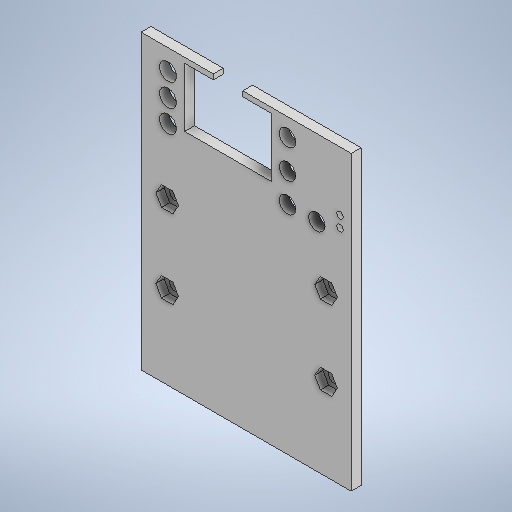
# Autodesk Inventor part: TES_Controller_V1_Case_Top
Saved by Autodesk Inventor 2025 (Build 290162000, 162)
## iProperties
Created: 2025-08-31
Part Number: TES_Controller_V1_Case_Top
Material: 常规
Document SubType Name: Modeling
Designer: 95052
Density: 1 g/cm^3
Appearance: 默认
Author: 95052
Autodesk Inventor part; units mm, degrees
ref_plane "YZ Plane" through (0, 0, 0) normal (1, 0, 0) x (0, 1, 0)
ref_plane "XZ Plane" through (0, 0, 0) normal (0, 1, 0) x (-1, 0, 0)
ref_plane "XY Plane" through (0, 0, 0) normal (0, 0, 1) x (1, 0, 0)
sketch "草图22" plane through (0, 0, 0) normal (0, 0, 1) x (1, 0, 0)
  line L0 (32.055, -44.6465) -> (-32.055, -44.6465)
  line L1 (-32.055, -44.6465) -> (-32.055, 44.6465)
  line L2 (-32.055, 44.6465) -> (32.055, 44.6465)
  line L3 (32.055, 44.6465) -> (32.055, -44.6465)
  line L4 (32.055, -44.6465) -> (-32.055, 44.6465) construction
  line L5 (-32.055, -44.6465) -> (32.055, 44.6465) construction
  line L6 (24.394, -19.5595) -> (-24.107, -19.5595) construction
  line L7 (-24.107, -19.5595) -> (-24.107, 4.4405) construction
  line L8 (-24.107, 4.4405) -> (24.394, 4.4405) construction
  line L9 (24.394, 4.4405) -> (24.394, -19.5595) construction
  line L10 (24.394, -19.5595) -> (-24.107, 4.4405) construction
  line L11 (-24.107, -19.5595) -> (24.394, 4.4405) construction
  circle A0 centre (-24.107, 4.4405) radius 1.7
  circle A1 centre (-24.107, -19.5595) radius 1.7
  circle A2 centre (24.394, -19.5595) radius 1.7
  circle A3 centre (24.394, 4.4405) radius 1.7
  point P0 (0, 0)
  point P1 (-14.525, 44.6465)
  point P2 (3.476, 44.6465)
  point P3 (0.1435, -7.5595)
  dimension "d101" = 89.293
  dimension "d102" = 64.11
  dimension "d103" = 7.661
  dimension "d104" = 7.948
  dimension "d105" = 25.087
  dimension "d106" = 40.206
  dimension "d107" = 17.53
  dimension "d108" = 28.579
  dimension "d109" = 3.4
  dimension "d110" = 3.4
  dimension "d111" = 3.4
  dimension "d112" = 3.4
  constraints: 24 end point, 4 centre point, 4 coincident, 4 midpoint, 4 parallel, 2 horizontal, 2 perpendicular, 2 point on line
  measures "d101" distance of L2.end L0.start
  measures "d102" distance of L0.start L0.end
  measures "d103" distance between parallel lines of L3 L9
  measures "d104" distance between parallel lines of L1 L7
  measures "d105" distance between parallel lines of L0 L6
  measures "d106" distance between parallel lines of L2 L8
  measures "d107" distance from line of L1 point (-14.525, 44.646)
  measures "d108" distance from line of L3 point (3.476, 44.646)
  measures "d109" diameter of A0
  measures "d110" diameter of A1
  measures "d111" diameter of A2
  measures "d112" diameter of A3
extrude "拉伸18" add sketch "草图22" along normal blind 0.5
sketch "草图23" plane through (0, 0, 0.5) normal (0, 0, 1) x (1, 0, 0)
  circle A0 centre (-24.107, 4.4405) radius 1.7 projected
  circle A1 centre (24.394, 4.4405) radius 1.7 projected
  circle A2 centre (24.394, -19.5595) radius 1.7 projected
  circle A3 centre (-24.107, -19.5595) radius 1.7 projected
  line L0 (-22.3749, -16.5595) -> (-20.6429, -19.5595)
  line L1 (-20.6429, -19.5595) -> (-22.3749, -22.5595)
  line L2 (-22.3749, -22.5595) -> (-25.8391, -22.5595)
  line L3 (-25.8391, -22.5595) -> (-27.5711, -19.5595)
  line L4 (-27.5711, -19.5595) -> (-25.8391, -16.5595)
  line L5 (-25.8391, -16.5595) -> (-22.3749, -16.5595)
  line L6 (-25.8391, 1.4405) -> (-27.5711, 4.4405)
  line L7 (-27.5711, 4.4405) -> (-25.8391, 7.4405)
  line L8 (-25.8391, 7.4405) -> (-22.3749, 7.4405)
  line L9 (-22.3749, 7.4405) -> (-20.6429, 4.4405)
  line L10 (-20.6429, 4.4405) -> (-22.3749, 1.4405)
  line L11 (-22.3749, 1.4405) -> (-25.8391, 1.4405)
  line L12 (22.6619, 1.4405) -> (20.9299, 4.4405)
  line L13 (20.9299, 4.4405) -> (22.6619, 7.4405)
  line L14 (22.6619, 7.4405) -> (26.1261, 7.4405)
  line L15 (26.1261, 7.4405) -> (27.8581, 4.4405)
  line L16 (27.8581, 4.4405) -> (26.1261, 1.4405)
  line L17 (26.1261, 1.4405) -> (22.6619, 1.4405)
  line L18 (22.6619, -22.5595) -> (20.9299, -19.5595)
  line L19 (20.9299, -19.5595) -> (22.6619, -16.5595)
  line L20 (22.6619, -16.5595) -> (26.1261, -16.5595)
  line L21 (26.1261, -16.5595) -> (27.8581, -19.5595)
  line L22 (27.8581, -19.5595) -> (26.1261, -22.5595)
  line L23 (26.1261, -22.5595) -> (22.6619, -22.5595)
  line L24 (32.055, 44.6465) -> (-32.055, 44.6465) projected
  line L25 (-32.055, -44.6465) -> (32.055, -44.6465) projected
  line L26 (-32.055, 44.6465) -> (32.055, 44.6465)
  line L27 (32.055, 44.6465) -> (32.055, -44.6465)
  line L28 (32.055, -44.6465) -> (-32.055, -44.6465)
  line L29 (-32.055, -44.6465) -> (-32.055, 44.6465)
  point P0 (0, 0)
  dimension "d115" = 6
  dimension "d116" = 6
  dimension "d117" = 6
  dimension "d118" = 6
  constraints: 56 end point, 4 coincident, 2 parallel, 1 horizontal, 1 perpendicular, 52 other
  measures "d115" distance between parallel lines of L5 L2
  measures "d116" distance between parallel lines of L11 L8
  measures "d117" distance between parallel lines of L17 L14
  measures "d118" distance between parallel lines of L23 L20
extrude "拉伸19" add sketch "草图23" along normal blind 2.5 contours L27 L25 L29 L24
sketch "草图24" plane through (0, 0, 0) normal (0, 0, -1) x (-1, 0, 0)
  circle A0 centre (-24.394, -19.5595) radius 1.7 projected
  circle A1 centre (-24.394, 4.4405) radius 1.7 projected
  line L0 (-26.1261, -16.5595) -> (-22.6619, -16.5595) projected
  line L1 (-22.6619, -16.5595) -> (-20.9299, -19.5595)
  line L2 (-20.9299, -19.5595) -> (-22.6619, -22.5595)
  line L3 (-22.6619, -22.5595) -> (-26.1261, -22.5595)
  line L4 (-26.1261, -22.5595) -> (-27.8581, -19.5595)
  line L5 (-27.8581, -19.5595) -> (-26.1261, -16.5595)
  line L6 (-26.1261, -16.5595) -> (-22.6619, -16.5595)
  line L7 (-22.6619, 1.4405) -> (-26.1261, 1.4405) projected
  line L8 (-26.1261, 1.4405) -> (-27.8581, 4.4405)
  line L9 (-27.8581, 4.4405) -> (-26.1261, 7.4405)
  line L10 (-26.1261, 7.4405) -> (-22.6619, 7.4405)
  line L11 (-22.6619, 7.4405) -> (-20.9299, 4.4405)
  line L12 (-20.9299, 4.4405) -> (-22.6619, 1.4405)
  line L13 (-22.6619, 1.4405) -> (-26.1261, 1.4405)
  circle A2 centre (24.107, 4.4405) radius 1.7 projected
  line L14 (22.3749, 1.4405) -> (20.6429, 4.4405)
  line L15 (20.6429, 4.4405) -> (22.3749, 7.4405)
  line L16 (22.3749, 7.4405) -> (25.8391, 7.4405)
  line L17 (25.8391, 7.4405) -> (27.5711, 4.4405)
  line L18 (27.5711, 4.4405) -> (25.8391, 1.4405)
  line L19 (25.8391, 1.4405) -> (22.3749, 1.4405)
  line L20 (25.8391, -16.5595) -> (27.5711, -19.5595)
  line L21 (27.5711, -19.5595) -> (25.8391, -22.5595)
  line L22 (25.8391, -22.5595) -> (22.3749, -22.5595)
  line L23 (22.3749, -22.5595) -> (20.6429, -19.5595)
  line L24 (20.6429, -19.5595) -> (22.3749, -16.5595)
  line L25 (22.3749, -16.5595) -> (25.8391, -16.5595)
  circle A3 centre (24.107, -19.5595) radius 1.7 projected
  point P0 (0, 0)
  point P1 (-24.394, -16.5595)
  point P2 (-24.394, 1.4405)
  point P3 (24.107, 1.4405)
  point P4 (24.107, -19.5595)
  point P5 (24.107, -16.5595)
  constraints: 48 end point, 6 midpoint, 3 coincident, 2 point on line, 52 other
extrude "拉伸20" add sketch "草图24" along normal blind 3
sketch "草图25" plane through (0, 0, 3) normal (0, 0, 1) x (1, 0, 0)
  circle A0 centre (-23.869, 38.3445) radius 2.6
  circle A1 centre (-23.869, 31.3595) radius 2.6
  circle A2 centre (-23.869, 24.5015) radius 2.6
  line L0 (32.055, 44.6465) -> (-32.055, 44.6465) projected
  line L1 (-32.055, 44.6465) -> (-32.055, -44.6465) projected
  circle A3 centre (12.608, 39.1095) radius 2.5
  line L2 (32.055, -44.6465) -> (32.055, 44.6465) projected
  circle A4 centre (12.608, 30.2185) radius 2.5
  circle A5 centre (12.608, 21.3885) radius 2.5
  circle A6 centre (21.582, 21.3885) radius 2.5
  circle A7 centre (28.639, 26.6255) radius 1
  circle A8 centre (28.639, 23.2155) radius 1
  line L3 (7.225, 20.5575) -> (-18.275, 20.5575) construction
  line L4 (-18.275, 20.5575) -> (-18.275, 47.0575) construction
  line L5 (-18.275, 47.0575) -> (7.225, 47.0575) construction
  line L6 (7.225, 47.0575) -> (7.225, 20.5575) construction
  line L7 (-18.775, 25.0575) -> (7.725, 25.0575)
  line L8 (7.725, 25.0575) -> (7.725, 43.0575)
  line L9 (-18.775, 43.0575) -> (-18.775, 25.0575)
  line L10 (-10.025, 43.0575) -> (-10.025, 47.0575)
  line L11 (-10.025, 47.0575) -> (-5.525, 47.0575)
  line L12 (-1.025, 43.0575) -> (-1.025, 47.0575)
  line L13 (-1.025, 47.0575) -> (-5.525, 47.0575)
  line L14 (7.725, 43.0575) -> (-1.025, 43.0575)
  line L15 (-10.025, 43.0575) -> (-18.775, 43.0575)
  point P0 (0, 0)
  point P1 (-5.525, 21.0575)
  point P2 (-5.525, 20.5575)
  dimension "d123" = 5.2
  dimension "d124" = 5.2
  dimension "d125" = 5.2
  dimension "d126" = 6.302
  dimension "d127" = 8.186
  dimension "d128" = 8.186
  dimension "d129" = 8.186
  dimension "d130" = 13.287
  dimension "d131" = 20.145
  dimension "d132" = 5.537
  dimension "d133" = 19.447
  dimension "d134" = 5
  dimension "d135" = 5
  dimension "d136" = 14.428
  dimension "d137" = 19.447
  dimension "d138" = 5
  dimension "d139" = 19.447
  dimension "d140" = 23.258
  dimension "d141" = 5
  dimension "d142" = 23.258
  dimension "d143" = 10.473
  dimension "d144" = 2
  dimension "d145" = 2
  dimension "d146" = 3.416
  dimension "d147" = 3.416
  dimension "d148" = 18.021
  dimension "d149" = 3.41
  dimension "d150" = 26.53
  dimension "d151" = 23.589
  dimension "d152" = 0.5
  dimension "d153" = 26.53
  dimension "d154" = 26.5
  dimension "d155" = 25.5
  dimension "d156" = 4.5
  dimension "d158" = 0.5
  dimension "d159" = 0.5
  constraints: 26 end point, 9 centre point, 5 parallel, 2 collinear, 2 horizontal, 2 perpendicular, 1 midpoint
  measures "d123" diameter of A0
  measures "d124" diameter of A1
  measures "d125" diameter of A2
  measures "d126" distance from line of L0 A0.centre
  measures "d127" distance from line of L1 A0.centre
  measures "d128" distance from line of L1 A1.centre
  measures "d129" distance from line of L1 A2.centre
  measures "d130" distance from line of L0 A1.centre
  measures "d131" distance from line of L0 A2.centre
  measures "d132" distance from line of L0 A3.centre
  measures "d133" distance from line of L2 A3.centre
  measures "d134" diameter of A3
  measures "d135" diameter of A4
  measures "d136" distance from line of L0 A4.centre
  measures "d137" distance from line of L2 A4.centre
  measures "d138" diameter of A5
  measures "d139" distance from line of L2 A5.centre
  measures "d140" distance from line of L0 A5.centre
  measures "d141" diameter of A6
  measures "d142" distance from line of L0 A6.centre
  measures "d143" distance from line of L2 A6.centre
  measures "d144" diameter of A7
  measures "d145" diameter of A8
  measures "d146" distance from line of L2 A7.centre
  measures "d147" distance from line of L2 A8.centre
  measures "d148" distance from line of L0 A7.centre
  measures "d149" distance of A7.centre A8.centre
  measures "d150" distance from line of L1 point (-5.525, 21.058)
  measures "d151" distance from line of L0 point (-5.525, 21.058)
  measures "d152" distance from line of point (-5.525, 21.058) L3
  measures "d153" distance from line of L1 point (-5.525, 20.558)
  measures "d154" distance of L3.end L4.end
  measures "d155" distance of L3.start L3.end
  measures "d156" distance between parallel lines of L3 L7
  measures "d158" distance between parallel lines of L4 L9
  measures "d159" distance between parallel lines of L6 L8
extrude "拉伸21" cut sketch "草图25" against normal up to next
